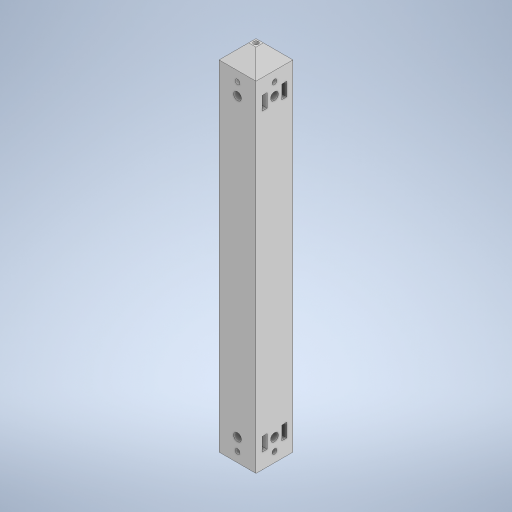
# Autodesk Inventor part: tensegrity_bar_4c_2base_frame
Saved by Autodesk Inventor 2023 (Build 270158000, 158)
## iProperties
Created: 2023-11-10
Part Number: tensegrity_bar_4c_2base_frame
Material: Všeobecné
Document SubType Name: Modeling
Designer: zavrel
Density: 1 g/cm^3
Appearance: Výchozí
Author: zavrel
Autodesk Inventor part; units mm, degrees
ref_plane "YZ Plane" through (0, 0, 0) normal (1, 0, 0) x (0, 1, 0)
ref_plane "XZ Plane" through (0, 0, 0) normal (0, 1, 0) x (-1, 0, 0)
ref_plane "XY Plane" through (0, 0, 0) normal (0, 0, 1) x (1, 0, 0)
sketch "Náčrt1" plane through (0, 0, 0) normal (0, 1, 0) x (-1, 0, 0)
  line L0 (0, 0) -> (15, 0)
  line L1 (15, 0) -> (15, -15)
  line L2 (15, -15) -> (0, -15)
  line L3 (0, -15) -> (0, 0)
  dimension "d0" = 15
  constraints: 8 end point, 2 parallel, 2 perpendicular, 1 horizontal
  measures "d0" distance of L0.end L1.end
extrude "Vysunutí1" add sketch "Náčrt1" along normal blind 150
sketch "Náčrt2" plane through (0, 150, 0) normal (0, 1, 0) x (1, 0, 0)
  line L0 (0, 15) -> (-15, 15) projected
  line L1 (-15, 15) -> (-15, 0) projected
  line L2 (-15, 0) -> (0, 0) projected
  line L3 (0, 0) -> (0, 15) projected
  circle A0 centre (-7.5, 7.5) radius 1
  line L4 (-15, 0) -> (0, 15) construction
  line L5 (-15, 15) -> (0, 0) construction
  point P0 (-7.5, 7.5)
  dimension "d3" = 2
  constraints: 4 end point, 1 centre point, 1 coincident, 1 midpoint, 1 perpendicular
  measures "d3" diameter of A0
extrude "Vysunutí2" cut sketch "Náčrt2" against normal through all contours A0
sketch "Náčrt3" plane through (0, 0, 0) normal (1, 0, 0) x (0, 0, -1)
  line L0 (0, 0) -> (15, 0) projected
  line L1 (15, 0) -> (15, 150) projected
  line L2 (0, 150) -> (15, 150) projected
  line L3 (0, 0) -> (0, 150) projected
  line L4 (7.5, 150) -> (7.5, 0) construction
  line L5 (15, 0) -> (0, 0) construction
  circle A0 centre (7.5, 135) radius 1.6
  circle A1 centre (7.5, 15) radius 1.6
  circle A2 centre (7.5, 140) radius 1
  circle A3 centre (7.5, 10) radius 1
  dimension "d6" = 3.2
  dimension "d7" = 15
  dimension "d8" = 15
  dimension "d16" = 2
  dimension "d17" = 10
  dimension "d18" = 10
  constraints: 4 centre point, 4 point on line, 2 end point, 2 equal radius, 2 midpoint
  measures "d6" diameter of A0
  measures "d7" distance from line of L2 A0.centre
  measures "d8" distance from line of L0 A1.centre
  measures "d16" diameter of A2
  measures "d17" distance from line of L2 A2.centre
  measures "d18" distance from line of L0 A3.centre
extrude "Vysunutí3" cut sketch "Náčrt3" against normal through all contours A0 | A1 | A2 | A3
sketch "Náčrt4" plane through (-15, 0, 0) normal (0, 0, 1) x (1, 0, 0)
  line L0 (0, 0) -> (15, 0) projected
  line L1 (15, 0) -> (15, 150) projected
  line L2 (0, 150) -> (15, 150) projected
  line L3 (0, 0) -> (0, 150) projected
  line L4 (6.5, 150) -> (8.5, 150) construction
  line L5 (7.5, 150) -> (7.5, 0) construction
  line L6 (8.5, 0) -> (6.5, 0) construction
  circle A0 centre (7.5, 135) radius 1.6
  circle A1 centre (7.5, 15) radius 1.6
  circle A2 centre (7.5, 140) radius 1
  circle A3 centre (7.5, 10) radius 1
  dimension "d11" = 3.2
  dimension "d12" = 15
  dimension "d13" = 15
  dimension "d19" = 2
  dimension "d20" = 10
  dimension "d21" = 10
  constraints: 4 centre point, 4 point on line, 2 end point, 2 equal radius, 2 midpoint
  measures "d11" diameter of A0
  measures "d12" distance from line of L2 A0.centre
  measures "d13" distance from line of L0 A1.centre
  measures "d19" diameter of A2
  measures "d20" distance from line of L2 A2.centre
  measures "d21" distance from line of L0 A3.centre
extrude "Vysunutí4" cut sketch "Náčrt4" against normal through all contours A0 | A1 | A2 | A3
sketch "Náčrt5" plane through (0, 0, 0) normal (1, 0, 0) x (0, 0, -1)
  circle A0 centre (7.5, 135) radius 1.6 projected
  circle A1 centre (7.5, 10) radius 1 projected
  circle A2 centre (7.5, 15) radius 1.6 projected
  circle A3 centre (7.5, 140) radius 1 projected
  line L0 (0, 0) -> (15, 0) projected
  line L1 (15, 0) -> (15, 150) projected
  line L2 (0, 150) -> (15, 150) projected
  line L3 (0, 0) -> (0, 150) projected
  line L4 (10.5, 137.75) -> (12.5, 137.75)
  line L5 (12.5, 137.75) -> (12.5, 132.25)
  line L6 (12.5, 132.25) -> (10.5, 132.25)
  line L7 (10.5, 132.25) -> (10.5, 137.75)
  circle A4 centre (7.5, 135) radius 1.6 construction
  line L8 (7.5, 135) -> (28.4763, 135) construction
  line L9 (15, 0) -> (15, 150) construction
  line L10 (15, 75) -> (0, 75) construction
  line L11 (0, 0) -> (0, 150) construction
  line L12 (10.5, 12.25) -> (12.5, 12.25)
  line L13 (12.5, 12.25) -> (12.5, 17.75)
  line L14 (12.5, 17.75) -> (10.5, 17.75)
  line L15 (10.5, 17.75) -> (10.5, 12.25)
  line L16 (6.5, 150) -> (8.5, 150) construction
  line L17 (7.5, 150) -> (7.5, 75) construction
  line L18 (4.5, 137.75) -> (2.5, 137.75)
  line L19 (2.5, 137.75) -> (2.5, 132.25)
  line L20 (2.5, 132.25) -> (4.5, 132.25)
  line L21 (4.5, 132.25) -> (4.5, 137.75)
  line L22 (2.5, 17.75) -> (4.5, 17.75)
  line L23 (4.5, 12.25) -> (2.5, 12.25)
  line L24 (2.5, 12.25) -> (2.5, 17.75)
  line L25 (4.5, 17.75) -> (4.5, 12.25)
  point P0 (12.5, 135)
  point P1 (12.5, 15)
  point P2 (11.5, 132.25)
  point P3 (11.5, 137.75)
  point P4 (2.5, 135)
  point P5 (2.5, 15)
  point P6 (3.5, 132.25)
  point P7 (3.5, 137.75)
  dimension "d25" = 2
  dimension "d26" = 2.5
  dimension "d27" = 5.5
  constraints: 38 end point, 17 symmetric about line, 7 midpoint, 2 horizontal, 2 parallel, 1 perpendicular, 1 point on line
  measures "d25" distance between parallel lines of L5 L7
  measures "d26" distance from line of L1 point (12.5, 135)
  measures "d27" distance of point (11.5, 132.25) point (11.5, 137.75)
extrude "Vysunutí5" cut sketch "Náčrt5" against normal blind 10.5 contours L4 L5 L6 L7 | L15 L14 L13 L12 | L21 L20 L19 L18 | L22 L25 L23 L24
sketch "Náčrt6" plane through (0, 0, -15) normal (0, 0, -1) x (-1, 0, 0)
  circle A0 centre (7.5, 135) radius 1.6 projected
  circle A1 centre (7.5, 140) radius 1 projected
  circle A2 centre (7.5, 15) radius 1.6 projected
  circle A3 centre (7.5, 10) radius 1 projected
  line L0 (0, 0) -> (15, 0) projected
  line L1 (15, 0) -> (15, 150) projected
  line L2 (0, 150) -> (15, 150) projected
  line L3 (0, 0) -> (0, 150) projected
  line L4 (12.5, 137.75) -> (10.5, 137.75)
  line L5 (10.5, 137.75) -> (10.5, 132.25)
  line L6 (10.5, 132.25) -> (12.5, 132.25)
  line L7 (12.5, 132.25) -> (12.5, 137.75)
  circle A4 centre (7.5, 135) radius 1.6 construction
  line L8 (7.5, 135) -> (15, 135) construction
  line L9 (0, 75) -> (15, 75) construction
  line L10 (12.5, 12.25) -> (10.5, 12.25)
  line L11 (10.5, 12.25) -> (10.5, 17.75)
  line L12 (10.5, 17.75) -> (12.5, 17.75)
  line L13 (12.5, 17.75) -> (12.5, 12.25)
  line L14 (7.5, 0) -> (7.5, 150) construction
  line L15 (2.5, 137.75) -> (4.5, 137.75)
  line L16 (4.5, 137.75) -> (4.5, 132.25)
  line L17 (4.5, 132.25) -> (2.5, 132.25)
  line L18 (2.5, 132.25) -> (2.5, 137.75)
  line L19 (4.5, 17.75) -> (2.5, 17.75)
  line L20 (4.5, 12.25) -> (4.5, 17.75)
  line L21 (2.5, 17.75) -> (2.5, 12.25)
  line L22 (2.5, 12.25) -> (4.5, 12.25)
  point P0 (12.5, 135)
  point P1 (12.5, 15)
  point P2 (2.5, 135)
  point P3 (2.5, 15)
  dimension "d30" = 2.5
  dimension "d31" = 2
  dimension "d32" = 5.5
  constraints: 38 end point, 15 symmetric about line, 5 midpoint, 2 parallel, 2 perpendicular, 2 point on line, 1 horizontal
  measures "d30" distance between parallel lines of L1 L7
  measures "d31" distance between parallel lines of L7 L5
  measures "d32" distance between parallel lines of L6 L4
extrude "Vysunutí6" cut sketch "Náčrt6" against normal blind 10.5 contours L7 L6 L5 L4 | L10 L11 L12 L13 | L15 L16 L17 L18 | L20 L22 L21 L19
chamfer "Zkosení2" distance 6 angle 45 8 edges at (-7.5, 0, -15) (0, 0, -7.5) (-15, 0, -7.5) (-7.5, 0, 0) (0, 150, -7.5) (-7.5, 150, -15) (-15, 150, -7.5) (-7.5, 150, 0)
